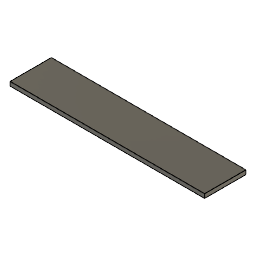
display_cover (Autodesk Fusion 360 design; units mm, degrees)
part number: 2026-03-18-20-37-46-438
Autodesk Fusion 360 part; units mm, degrees
sketch "Sketch1" plane through (0, 0, 0) normal (0, 0, 1) x (1, 0, 0)
  line L0 (0, 0) -> (94, 0)
  line L1 (94, 0) -> (94, -25)
  line L2 (94, -25) -> (0, -25)
  line L3 (0, -25) -> (0, 0)
  dimension "d1" = 94
  dimension "d2" = 25
  constraint horizontal L0
  constraint vertical L1
  constraint horizontal L2
  constraint vertical L3
  constraint coincident L0.start L3.end
  measures "d1" distance of L0.start L0.end
  measures "d2" distance of L0.start L2.end
extrude "Extrude1" add sketch "Sketch1" along normal blind 2
extrude "Extrude2" cut 1 faces at (62.6667, -25, 0.6667) along direction (0, 1, 0) blind 2.7
extrude "Extrude3" cut 1 faces at (62.6667, -22.3, 0.6667) along direction (0, 1, 0) blind 1.7
extrude "Extrude4" cut 1 faces at (62.6667, -20.6, 0.6667) along direction (0, 1, 0) blind 1
extrude "Extrude5" add 1 faces at (62.6667, -19.6, 0.6667) along direction (0, -1, 0) blind 0.4
